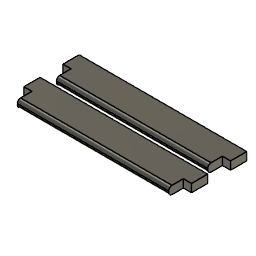
card-shuffler (Autodesk Fusion 360 archive; units mm, degrees)
design "card-shuffler-gates"
part number: 2026-07-29-22-33-21-616
part number: 2026-07-29-22-39-06-031
part number: 2026-07-29-22-39-06-037
Autodesk Fusion 360 part; units mm, degrees
(part 1 of 8)
sketch "Sketch1" plane through (0, 0, 0) normal (0, 0, 1) x (1, 0, 0)
  line L0 (0, 0) -> (93, 0)
  line L1 (93, 0) -> (93, -19)
  line L2 (93, -19) -> (0, -19)
  line L3 (0, -19) -> (0, 0)
  line L4 (0, 0) -> (-5, 0)
  line L5 (-5, 0) -> (-5, -10)
  line L6 (-5, -10) -> (0, -10)
  line L7 (0, -10) -> (0, 0)
  line L8 (93, 0) -> (98, 0)
  line L9 (98, 0) -> (98, -10)
  line L10 (98, -10) -> (93, -10)
  line L11 (93, -10) -> (93, 0)
  dimension "d1" = 93
  dimension "d2" = 19
  constraint horizontal L0
  constraint vertical L1
  constraint horizontal L2
  constraint vertical L3
  constraint coincident L0.start L3.end
  constraint horizontal L4
  constraint vertical L5
  constraint horizontal L6
  constraint vertical L7
  constraint horizontal L8
  constraint vertical L9
  constraint horizontal L10
  constraint vertical L11
  measures "d1" distance of L0.start L0.end
  measures "d2" distance of L0.start L2.end
extrude "Extrude1" add sketch "Sketch1" along normal blind 5 makes body 1
copy_body "CopyPasteBodies1" bodies 1 makes body 2
move_body "Move1" bodies 2 to x (1, 0, 0) y (0, 1, 0) z (0, 0, 1) at (0, 24, 0)
copy_body "Body->Comp1" bodies 1 removing the originals makes body 3 in component "Component"
copy_body "Body->Comp2" bodies 2 removing the originals makes body 4 in component "Component'"
fillet "Fillet1" radius 2 2 edges at (46.5, 5, 0) (46.5, 5, 5) on bodies 4 in component "Component'"
fillet "Fillet1'" radius 2 2 edges at (46.5, -19, 5) (46.5, -19, 0) on bodies 3 in component "Component"
component "Component" placed x (1, 0, 0) y (0, 1, 0) z (0, 0, 1) at (0, 0, 0)
component "Component'" placed x (1, 0, 0) y (0, 1, 0) z (0, 0, 1) at (0, 0, 0)
equation "d2 = 10 mm + 9 mm"

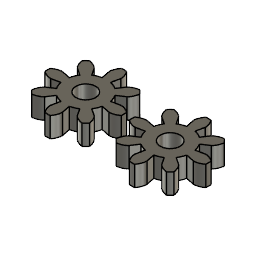
design "card-shuffler-driven-gears"
part number: 2026-07-29-20-17-55-869
part number: 2026-07-29-23-17-52-901
Autodesk Fusion 360 part; units mm, degrees
sketch "Sketch1" plane through (0, 0, 6) normal (0, 0, 1) x (-1, 0, 0)
  arc A0 (-4.7736, 3.1514) -> (-5.6038, 1.147) centre (0, 0) ccw
  line L0 (-5.6038, 1.147) -> (-7.8914, 1.6152)
  line L1 (-7.8914, 1.6152) -> (-7.8925, 1.6154)
  spline S0 degree 5 poles (-7.8925, 1.6154) (-7.8926, 1.6155) (-7.8929, 1.6155) (-7.8933, 1.6156) (-7.8941, 1.6157) (-7.8951, 1.6159) (-7.8964, 1.6161) (-7.8978, 1.6164) (-7.8993, 1.6166) (-7.9011, 1.6169) (-7.9029, 1.6172) (-7.905, 1.6175) (-7.9072, 1.6178) (-7.9095, 1.6181) (-7.912, 1.6184) (-7.9146, 1.6188) (-7.9174, 1.6191) (-7.9204, 1.6195) (-7.9234, 1.6198) (-7.9266, 1.6202) (-7.93, 1.6205) (-7.9334, 1.6209) (-7.9371, 1.6212) (-7.9408, 1.6216) (-7.9447, 1.6219) (-7.9487, 1.6223) (-7.9528, 1.6226) (-7.957, 1.6229) (-7.9614, 1.6232) (-7.9659, 1.6235) (-7.9705, 1.6238) (-7.9752, 1.6241) (-7.9801, 1.6244) (-7.985, 1.6246) (-7.9901, 1.6249) (-7.9953, 1.6251) (-8.0006, 1.6253) (-8.006, 1.6255) (-8.0115, 1.6257) (-8.0171, 1.6258) (-8.0229, 1.6259) (-8.0287, 1.626) (-8.0346, 1.6261) (-8.0407, 1.6262) (-8.0468, 1.6262) (-8.0531, 1.6263) (-8.0594, 1.6263) (-8.0659, 1.6262) (-8.0724, 1.6262) (-8.079, 1.6261) (-8.0858, 1.626) (-8.0926, 1.6258) (-8.0995, 1.6257) (-8.1065, 1.6255) (-8.1136, 1.6253) (-8.1208, 1.625) (-8.1281, 1.6247) (-8.1355, 1.6244) (-8.143, 1.6241) (-8.1505, 1.6237) (-8.1581, 1.6233) (-8.1658, 1.6228) (-8.1737, 1.6223) (-8.1815, 1.6218) (-8.1895, 1.6213) (-8.1976, 1.6207) (-8.2057, 1.6201) (-8.2139, 1.6194) (-8.2222, 1.6187) (-8.2306, 1.618) (-8.239, 1.6172) (-8.2475, 1.6164) (-8.2561, 1.6156) (-8.2648, 1.6147) (-8.2735, 1.6138) (-8.2824, 1.6128) (-8.2913, 1.6118) (-8.3002, 1.6108) (-8.3093, 1.6097) (-8.3184, 1.6086) (-8.3276, 1.6074) (-8.3368, 1.6062) (-8.3461, 1.605) (-8.3555, 1.6037) (-8.365, 1.6024) (-8.3745, 1.601) (-8.3841, 1.5996) (-8.3937, 1.5981) (-8.4035, 1.5966) (-8.4132, 1.5951) (-8.4231, 1.5935) (-8.433, 1.5918) (-8.443, 1.5901) (-8.453, 1.5884) (-8.4631, 1.5866) (-8.4733, 1.5848) (-8.4835, 1.5829) (-8.4938, 1.581) (-8.5041, 1.5791) (-8.5145, 1.577) (-8.525, 1.575) (-8.5355, 1.5729) (-8.546, 1.5707) (-8.5567, 1.5685) (-8.5673, 1.5663) (-8.5781, 1.564) (-8.5889, 1.5616) (-8.5997, 1.5592) (-8.6106, 1.5568) (-8.6215, 1.5543) (-8.6325, 1.5517) (-8.6436, 1.5492) (-8.6547, 1.5465) (-8.6659, 1.5438) (-8.6771, 1.5411) (-8.6883, 1.5383) (-8.6996, 1.5354) (-8.711, 1.5325) (-8.7224, 1.5296) (-8.7338, 1.5266) (-8.7453, 1.5235) (-8.7569, 1.5204) (-8.7684, 1.5173) (-8.7801, 1.514) (-8.7918, 1.5108) (-8.8035, 1.5075) (-8.8153, 1.5041) (-8.8271, 1.5007) (-8.8389, 1.4972) (-8.8508, 1.4937) (-8.8628, 1.4901) (-8.8747, 1.4865) (-8.8868, 1.4828) (-8.8988, 1.479) (-8.9109, 1.4752) (-8.9231, 1.4714) (-8.9353, 1.4675) (-8.9475, 1.4635) (-8.9598, 1.4595) (-8.9721, 1.4554) (-8.9844, 1.4513) (-8.9968, 1.4471) (-9.0092, 1.4429) (-9.0217, 1.4386) (-9.0342, 1.4343) (-9.0467, 1.4299) (-9.0593, 1.4254) (-9.0718, 1.4209) (-9.0845, 1.4163) (-9.0971, 1.4117) (-9.1098, 1.407) (-9.1226, 1.4023) (-9.1353, 1.3975) (-9.1481, 1.3927) (-9.161, 1.3877) (-9.1738, 1.3828) (-9.1867, 1.3778) (-9.1997, 1.3727) (-9.2126, 1.3676) (-9.2256, 1.3624) (-9.2386, 1.3571) (-9.2517, 1.3518) (-9.2647, 1.3465) (-9.2778, 1.3411) (-9.291, 1.3356) (-9.3041, 1.3301) (-9.3173, 1.3245) (-9.3305, 1.3188) (-9.3438, 1.3131) (-9.3571, 1.3074) (-9.3704, 1.3015) (-9.3837, 1.2957) (-9.397, 1.2897) (-9.4104, 1.2837) (-9.4238, 1.2777) (-9.4372, 1.2716) (-9.4507, 1.2654) (-9.4641, 1.2592) (-9.4776, 1.2529) (-9.4911, 1.2465) (-9.5047, 1.2401) (-9.5182, 1.2337) (-9.5318, 1.2272) (-9.5454, 1.2206) (-9.559, 1.214) (-9.5727, 1.2073) (-9.5863, 1.2005) (-9.6, 1.1937) (-9.6137, 1.1868) (-9.6275, 1.1799) (-9.6412, 1.1729) (-9.655, 1.1659) (-9.6687, 1.1588) (-9.6825, 1.1516) (-9.6964, 1.1444) (-9.7102, 1.1371) (-9.7241, 1.1298) (-9.7379, 1.1224) (-9.7518, 1.1149) (-9.7657, 1.1074) (-9.7796, 1.0998) (-9.7936, 1.0922) (-9.8075, 1.0845) (-9.8215, 1.0767) (-9.8355, 1.0689) (-9.8494, 1.061) (-9.8635, 1.0531) (-9.8775, 1.0451) (-9.8915, 1.037) (-9.9056, 1.0289) (-9.9196, 1.0207) (-9.9337, 1.0125) (-9.9478, 1.0042) (-9.9619, 0.9959) (-9.976, 0.9875) (-9.9901, 0.979) (-10.0042, 0.9705) (-10.0184, 0.9619) (-10.0325, 0.9532) (-10.0467, 0.9445) (-10.0608, 0.9357) (-10.075, 0.9269) (-10.0892, 0.918) (-10.1034, 0.9091) (-10.1176, 0.9001) (-10.1318, 0.891) (-10.1461, 0.8819) (-10.1603, 0.8727) (-10.1745, 0.8635) (-10.1888, 0.8542) (-10.203, 0.8448) (-10.2173, 0.8354) (-10.2316, 0.8259) (-10.2458, 0.8163) (-10.2601, 0.8067) (-10.2744, 0.7971) (-10.2887, 0.7874) (-10.303, 0.7776) (-10.3173, 0.7677) (-10.3316, 0.7578) (-10.3459, 0.7479) (-10.3573, 0.7399) (-10.3659, 0.7338) (-10.3716, 0.7298) (-10.3745, 0.7278) knots 0 0 0 0 0 0 0.00416667 0.00833333 0.0125 0.01666667 0.02083333 0.025 0.02916667 0.03333333 0.0375 0.04166667 0.04583333 0.05 0.05416667 0.05833333 0.0625 0.06666667 0.07083333 0.075 0.07916667 0.08333333 0.0875 0.09166667 0.09583333 0.1 0.10416667 0.10833333 0.1125 0.11666667 0.12083333 0.125 0.12916667 0.13333333 0.1375 0.14166667 0.14583333 0.15 0.15416667 0.15833333 0.1625 0.16666667 0.17083333 0.175 0.17916667 0.18333333 0.1875 0.19166667 0.19583333 0.2 0.20416667 0.20833333 0.2125 0.21666667 0.22083333 0.225 0.22916667 0.23333333 0.2375 0.24166667 0.24583333 0.25 0.25416667 0.25833333 0.2625 0.26666667 0.27083333 0.275 0.27916667 0.28333333 0.2875 0.29166667 0.29583333 0.3 0.30416667 0.30833333 0.3125 0.31666667 0.32083333 0.325 0.32916667 0.33333333 0.3375 0.34166667 0.34583333 0.35 0.35416667 0.35833333 0.3625 0.36666667 0.37083333 0.375 0.37916667 0.38333333 0.3875 0.39166667 0.39583333 0.4 0.40416667 0.40833333 0.4125 0.41666667 0.42083333 0.425 0.42916667 0.43333333 0.4375 0.44166667 0.44583333 0.45 0.45416667 0.45833333 0.4625 0.46666667 0.47083333 0.475 0.47916667 0.48333333 0.4875 0.49166667 0.49583333 0.5 0.50416667 0.50833333 0.5125 0.51666667 0.52083333 0.525 0.52916667 0.53333333 0.5375 0.54166667 0.54583333 0.55 0.55416667 0.55833333 0.5625 0.56666667 0.57083333 0.575 0.57916667 0.58333333 0.5875 0.59166667 0.59583333 0.6 0.60416667 0.60833333 0.6125 0.61666667 0.62083333 0.625 0.62916667 0.63333333 0.6375 0.64166667 0.64583333 0.65 0.65416667 0.65833333 0.6625 0.66666667 0.67083333 0.675 0.67916667 0.68333333 0.6875 0.69166667 0.69583333 0.7 0.70416667 0.70833333 0.7125 0.71666667 0.72083333 0.725 0.72916667 0.73333333 0.7375 0.74166667 0.74583333 0.75 0.75416667 0.75833333 0.7625 0.76666667 0.77083333 0.775 0.77916667 0.78333333 0.7875 0.79166667 0.79583333 0.8 0.80416667 0.80833333 0.8125 0.81666667 0.82083333 0.825 0.82916667 0.83333333 0.8375 0.84166667 0.84583333 0.85 0.85416667 0.85833333 0.8625 0.86666667 0.87083333 0.875 0.87916667 0.88333333 0.8875 0.89166667 0.89583333 0.9 0.90416667 0.90833333 0.9125 0.91666667 0.92083333 0.925 0.92916667 0.93333333 0.9375 0.94166667 0.94583333 0.95 0.95416667 0.95833333 0.9625 0.96666667 0.97083333 0.975 0.97916667 0.98333333 0.9875 0.99166667 0.99583333 1 1 1 1 1 1
  arc A1 (-10.3745, 0.7278) -> (-10.3745, -0.7278) centre (0, 0) ccw
  spline S1 degree 5 poles (-10.3745, -0.7278) (-10.3716, -0.7298) (-10.3659, -0.7338) (-10.3573, -0.7399) (-10.3459, -0.7479) (-10.3316, -0.7578) (-10.3173, -0.7677) (-10.303, -0.7776) (-10.2887, -0.7874) (-10.2744, -0.7971) (-10.2601, -0.8067) (-10.2458, -0.8163) (-10.2316, -0.8259) (-10.2173, -0.8354) (-10.203, -0.8448) (-10.1888, -0.8542) (-10.1745, -0.8635) (-10.1603, -0.8727) (-10.1461, -0.8819) (-10.1318, -0.891) (-10.1176, -0.9001) (-10.1034, -0.9091) (-10.0892, -0.918) (-10.075, -0.9269) (-10.0608, -0.9357) (-10.0467, -0.9445) (-10.0325, -0.9532) (-10.0184, -0.9619) (-10.0042, -0.9705) (-9.9901, -0.979) (-9.976, -0.9875) (-9.9619, -0.9959) (-9.9478, -1.0042) (-9.9337, -1.0125) (-9.9196, -1.0207) (-9.9056, -1.0289) (-9.8915, -1.037) (-9.8775, -1.0451) (-9.8635, -1.0531) (-9.8494, -1.061) (-9.8355, -1.0689) (-9.8215, -1.0767) (-9.8075, -1.0845) (-9.7936, -1.0922) (-9.7796, -1.0998) (-9.7657, -1.1074) (-9.7518, -1.1149) (-9.7379, -1.1224) (-9.7241, -1.1298) (-9.7102, -1.1371) (-9.6964, -1.1444) (-9.6825, -1.1516) (-9.6687, -1.1588) (-9.655, -1.1659) (-9.6412, -1.1729) (-9.6275, -1.1799) (-9.6137, -1.1868) (-9.6, -1.1937) (-9.5863, -1.2005) (-9.5727, -1.2073) (-9.559, -1.214) (-9.5454, -1.2206) (-9.5318, -1.2272) (-9.5182, -1.2337) (-9.5047, -1.2401) (-9.4911, -1.2465) (-9.4776, -1.2529) (-9.4641, -1.2592) (-9.4507, -1.2654) (-9.4372, -1.2716) (-9.4238, -1.2777) (-9.4104, -1.2837) (-9.397, -1.2897) (-9.3837, -1.2957) (-9.3704, -1.3015) (-9.3571, -1.3074) (-9.3438, -1.3131) (-9.3305, -1.3188) (-9.3173, -1.3245) (-9.3041, -1.3301) (-9.291, -1.3356) (-9.2778, -1.3411) (-9.2647, -1.3465) (-9.2517, -1.3518) (-9.2386, -1.3571) (-9.2256, -1.3624) (-9.2126, -1.3676) (-9.1997, -1.3727) (-9.1867, -1.3778) (-9.1738, -1.3828) (-9.161, -1.3877) (-9.1481, -1.3927) (-9.1353, -1.3975) (-9.1226, -1.4023) (-9.1098, -1.407) (-9.0971, -1.4117) (-9.0845, -1.4163) (-9.0718, -1.4209) (-9.0593, -1.4254) (-9.0467, -1.4299) (-9.0342, -1.4343) (-9.0217, -1.4386) (-9.0092, -1.4429) (-8.9968, -1.4471) (-8.9844, -1.4513) (-8.9721, -1.4554) (-8.9598, -1.4595) (-8.9475, -1.4635) (-8.9353, -1.4675) (-8.9231, -1.4714) (-8.9109, -1.4752) (-8.8988, -1.479) (-8.8868, -1.4828) (-8.8747, -1.4865) (-8.8628, -1.4901) (-8.8508, -1.4937) (-8.8389, -1.4972) (-8.8271, -1.5007) (-8.8153, -1.5041) (-8.8035, -1.5075) (-8.7918, -1.5108) (-8.7801, -1.514) (-8.7684, -1.5173) (-8.7569, -1.5204) (-8.7453, -1.5235) (-8.7338, -1.5266) (-8.7224, -1.5296) (-8.711, -1.5325) (-8.6996, -1.5354) (-8.6883, -1.5383) (-8.6771, -1.5411) (-8.6659, -1.5438) (-8.6547, -1.5465) (-8.6436, -1.5492) (-8.6325, -1.5517) (-8.6215, -1.5543) (-8.6106, -1.5568) (-8.5997, -1.5592) (-8.5889, -1.5616) (-8.5781, -1.564) (-8.5673, -1.5663) (-8.5567, -1.5685) (-8.546, -1.5707) (-8.5355, -1.5729) (-8.525, -1.575) (-8.5145, -1.577) (-8.5041, -1.5791) (-8.4938, -1.581) (-8.4835, -1.5829) (-8.4733, -1.5848) (-8.4631, -1.5866) (-8.453, -1.5884) (-8.443, -1.5901) (-8.433, -1.5918) (-8.4231, -1.5935) (-8.4132, -1.5951) (-8.4035, -1.5966) (-8.3937, -1.5981) (-8.3841, -1.5996) (-8.3745, -1.601) (-8.365, -1.6024) (-8.3555, -1.6037) (-8.3461, -1.605) (-8.3368, -1.6062) (-8.3276, -1.6074) (-8.3184, -1.6086) (-8.3093, -1.6097) (-8.3002, -1.6108) (-8.2913, -1.6118) (-8.2824, -1.6128) (-8.2735, -1.6138) (-8.2648, -1.6147) (-8.2561, -1.6156) (-8.2475, -1.6164) (-8.239, -1.6172) (-8.2306, -1.618) (-8.2222, -1.6187) (-8.2139, -1.6194) (-8.2057, -1.6201) (-8.1976, -1.6207) (-8.1895, -1.6213) (-8.1815, -1.6218) (-8.1737, -1.6223) (-8.1658, -1.6228) (-8.1581, -1.6233) (-8.1505, -1.6237) (-8.143, -1.6241) (-8.1355, -1.6244) (-8.1281, -1.6247) (-8.1208, -1.625) (-8.1136, -1.6253) (-8.1065, -1.6255) (-8.0995, -1.6257) (-8.0926, -1.6258) (-8.0858, -1.626) (-8.079, -1.6261) (-8.0724, -1.6262) (-8.0659, -1.6262) (-8.0594, -1.6263) (-8.0531, -1.6263) (-8.0468, -1.6262) (-8.0407, -1.6262) (-8.0346, -1.6261) (-8.0287, -1.626) (-8.0229, -1.6259) (-8.0171, -1.6258) (-8.0115, -1.6257) (-8.006, -1.6255) (-8.0006, -1.6253) (-7.9953, -1.6251) (-7.9901, -1.6249) (-7.985, -1.6246) (-7.9801, -1.6244) (-7.9752, -1.6241) (-7.9705, -1.6238) (-7.9659, -1.6235) (-7.9614, -1.6232) (-7.957, -1.6229) (-7.9528, -1.6226) (-7.9487, -1.6223) (-7.9447, -1.6219) (-7.9408, -1.6216) (-7.9371, -1.6212) (-7.9334, -1.6209) (-7.93, -1.6205) (-7.9266, -1.6202) (-7.9234, -1.6198) (-7.9204, -1.6195) (-7.9174, -1.6191) (-7.9146, -1.6188) (-7.912, -1.6184) (-7.9095, -1.6181) (-7.9072, -1.6178) (-7.905, -1.6175) (-7.9029, -1.6172) (-7.9011, -1.6169) (-7.8993, -1.6166) (-7.8978, -1.6164) (-7.8964, -1.6161) (-7.8951, -1.6159) (-7.8941, -1.6157) (-7.8933, -1.6156) (-7.8929, -1.6155) (-7.8926, -1.6155) (-7.8925, -1.6154) knots -1 -1 -1 -1 -1 -1 -0.99583333 -0.99166667 -0.9875 -0.98333333 -0.97916667 -0.975 -0.97083333 -0.96666667 -0.9625 -0.95833333 -0.95416667 -0.95 -0.94583333 -0.94166667 -0.9375 -0.93333333 -0.92916667 -0.925 -0.92083333 -0.91666667 -0.9125 -0.90833333 -0.90416667 -0.9 -0.89583333 -0.89166667 -0.8875 -0.88333333 -0.87916667 -0.875 -0.87083333 -0.86666667 -0.8625 -0.85833333 -0.85416667 -0.85 -0.84583333 -0.84166667 -0.8375 -0.83333333 -0.82916667 -0.825 -0.82083333 -0.81666667 -0.8125 -0.80833333 -0.80416667 -0.8 -0.79583333 -0.79166667 -0.7875 -0.78333333 -0.77916667 -0.775 -0.77083333 -0.76666667 -0.7625 -0.75833333 -0.75416667 -0.75 -0.74583333 -0.74166667 -0.7375 -0.73333333 -0.72916667 -0.725 -0.72083333 -0.71666667 -0.7125 -0.70833333 -0.70416667 -0.7 -0.69583333 -0.69166667 -0.6875 -0.68333333 -0.67916667 -0.675 -0.67083333 -0.66666667 -0.6625 -0.65833333 -0.65416667 -0.65 -0.64583333 -0.64166667 -0.6375 -0.63333333 -0.62916667 -0.625 -0.62083333 -0.61666667 -0.6125 -0.60833333 -0.60416667 -0.6 -0.59583333 -0.59166667 -0.5875 -0.58333333 -0.57916667 -0.575 -0.57083333 -0.56666667 -0.5625 -0.55833333 -0.55416667 -0.55 -0.54583333 -0.54166667 -0.5375 -0.53333333 -0.52916667 -0.525 -0.52083333 -0.51666667 -0.5125 -0.50833333 -0.50416667 -0.5 -0.49583333 -0.49166667 -0.4875 -0.48333333 -0.47916667 -0.475 -0.47083333 -0.46666667 -0.4625 -0.45833333 -0.45416667 -0.45 -0.44583333 -0.44166667 -0.4375 -0.43333333 -0.42916667 -0.425 -0.42083333 -0.41666667 -0.4125 -0.40833333 -0.40416667 -0.4 -0.39583333 -0.39166667 -0.3875 -0.38333333 -0.37916667 -0.375 -0.37083333 -0.36666667 -0.3625 -0.35833333 -0.35416667 -0.35 -0.34583333 -0.34166667 -0.3375 -0.33333333 -0.32916667 -0.325 -0.32083333 -0.31666667 -0.3125 -0.30833333 -0.30416667 -0.3 -0.29583333 -0.29166667 -0.2875 -0.28333333 -0.27916667 -0.275 -0.27083333 -0.26666667 -0.2625 -0.25833333 -0.25416667 -0.25 -0.24583333 -0.24166667 -0.2375 -0.23333333 -0.22916667 -0.225 -0.22083333 -0.21666667 -0.2125 -0.20833333 -0.20416667 -0.2 -0.19583333 -0.19166667 -0.1875 -0.18333333 -0.17916667 -0.175 -0.17083333 -0.16666667 -0.1625 -0.15833333 -0.15416667 -0.15 -0.14583333 -0.14166667 -0.1375 -0.13333333 -0.12916667 -0.125 -0.12083333 -0.11666667 -0.1125 -0.10833333 -0.10416667 -0.1 -0.09583333 -0.09166667 -0.0875 -0.08333333 -0.07916667 -0.075 -0.07083333 -0.06666667 -0.0625 -0.05833333 -0.05416667 -0.05 -0.04583333 -0.04166667 -0.0375 -0.03333333 -0.02916667 -0.025 -0.02083333 -0.01666667 -0.0125 -0.00833333 -0.00416667 0 0 0 0 0 0
  line L2 (-7.8925, -1.6154) -> (-7.8914, -1.6152)
  line L3 (-7.8914, -1.6152) -> (-5.6038, -1.147)
  arc A2 (-5.6038, -1.147) -> (-4.7736, -3.1514) centre (0, 0) ccw
  line L4 (-4.7736, -3.1514) -> (-6.7222, -4.4379)
  line L5 (-6.7222, -4.4379) -> (-6.7231, -4.4385)
  spline S2 degree 5 poles (-6.7231, -4.4385) (-6.7232, -4.4386) (-6.7235, -4.4388) (-6.7238, -4.439) (-6.7244, -4.4394) (-6.7253, -4.4401) (-6.7263, -4.4408) (-6.7275, -4.4416) (-6.7288, -4.4425) (-6.7302, -4.4436) (-6.7317, -4.4447) (-6.7334, -4.4459) (-6.7352, -4.4473) (-6.737, -4.4487) (-6.739, -4.4502) (-6.7411, -4.4519) (-6.7434, -4.4536) (-6.7457, -4.4554) (-6.7481, -4.4573) (-6.7506, -4.4593) (-6.7532, -4.4614) (-6.7559, -4.4637) (-6.7587, -4.466) (-6.7616, -4.4684) (-6.7646, -4.4708) (-6.7677, -4.4734) (-6.7708, -4.4761) (-6.774, -4.4789) (-6.7774, -4.4818) (-6.7807, -4.4847) (-6.7842, -4.4878) (-6.7877, -4.4909) (-6.7914, -4.4942) (-6.7951, -4.4975) (-6.7988, -4.5009) (-6.8026, -4.5044) (-6.8065, -4.508) (-6.8105, -4.5117) (-6.8145, -4.5155) (-6.8186, -4.5194) (-6.8227, -4.5233) (-6.8269, -4.5274) (-6.8312, -4.5315) (-6.8355, -4.5357) (-6.8399, -4.54) (-6.8443, -4.5444) (-6.8488, -4.5489) (-6.8533, -4.5535) (-6.8579, -4.5582) (-6.8626, -4.5629) (-6.8672, -4.5678) (-6.872, -4.5727) (-6.8768, -4.5777) (-6.8816, -4.5828) (-6.8864, -4.588) (-6.8914, -4.5932) (-6.8963, -4.5986) (-6.9013, -4.604) (-6.9063, -4.6096) (-6.9114, -4.6152) (-6.9165, -4.6208) (-6.9216, -4.6266) (-6.9268, -4.6325) (-6.932, -4.6384) (-6.9373, -4.6444) (-6.9426, -4.6505) (-6.9479, -4.6567) (-6.9532, -4.663) (-6.9586, -4.6693) (-6.964, -4.6758) (-6.9694, -4.6823) (-6.9749, -4.6889) (-6.9804, -4.6956) (-6.9859, -4.7023) (-6.9914, -4.7092) (-6.997, -4.7161) (-7.0025, -4.7231) (-7.0082, -4.7301) (-7.0138, -4.7373) (-7.0194, -4.7445) (-7.0251, -4.7518) (-7.0308, -4.7592) (-7.0365, -4.7667) (-7.0422, -4.7743) (-7.048, -4.7819) (-7.0537, -4.7896) (-7.0595, -4.7974) (-7.0653, -4.8052) (-7.0711, -4.8132) (-7.0769, -4.8212) (-7.0828, -4.8293) (-7.0886, -4.8375) (-7.0945, -4.8457) (-7.1004, -4.854) (-7.1062, -4.8624) (-7.1121, -4.8709) (-7.118, -4.8794) (-7.1239, -4.8881) (-7.1299, -4.8968) (-7.1358, -4.9055) (-7.1417, -4.9144) (-7.1477, -4.9233) (-7.1536, -4.9323) (-7.1596, -4.9414) (-7.1655, -4.9505) (-7.1715, -4.9597) (-7.1775, -4.969) (-7.1834, -4.9784) (-7.1894, -4.9878) (-7.1954, -4.9973) (-7.2014, -5.0069) (-7.2074, -5.0165) (-7.2133, -5.0262) (-7.2193, -5.036) (-7.2253, -5.0459) (-7.2313, -5.0558) (-7.2373, -5.0658) (-7.2432, -5.0759) (-7.2492, -5.0861) (-7.2552, -5.0963) (-7.2612, -5.1066) (-7.2671, -5.1169) (-7.2731, -5.1274) (-7.279, -5.1379) (-7.285, -5.1484) (-7.2909, -5.1591) (-7.2969, -5.1698) (-7.3028, -5.1805) (-7.3087, -5.1914) (-7.3147, -5.2023) (-7.3206, -5.2133) (-7.3265, -5.2243) (-7.3324, -5.2354) (-7.3383, -5.2466) (-7.3441, -5.2578) (-7.35, -5.2692) (-7.3559, -5.2805) (-7.3617, -5.292) (-7.3675, -5.3035) (-7.3734, -5.3151) (-7.3792, -5.3267) (-7.385, -5.3384) (-7.3908, -5.3502) (-7.3965, -5.362) (-7.4023, -5.3739) (-7.408, -5.3859) (-7.4138, -5.3979) (-7.4195, -5.41) (-7.4252, -5.4222) (-7.4309, -5.4344) (-7.4366, -5.4467) (-7.4422, -5.4591) (-7.4478, -5.4715) (-7.4535, -5.484) (-7.4591, -5.4965) (-7.4647, -5.5091) (-7.4702, -5.5218) (-7.4758, -5.5345) (-7.4813, -5.5473) (-7.4868, -5.5601) (-7.4923, -5.5731) (-7.4978, -5.586) (-7.5033, -5.5991) (-7.5087, -5.6122) (-7.5141, -5.6253) (-7.5195, -5.6385) (-7.5249, -5.6518) (-7.5302, -5.6651) (-7.5356, -5.6785) (-7.5409, -5.692) (-7.5462, -5.7055) (-7.5514, -5.7191) (-7.5567, -5.7327) (-7.5619, -5.7464) (-7.5671, -5.7602) (-7.5722, -5.774) (-7.5774, -5.7878) (-7.5825, -5.8018) (-7.5876, -5.8158) (-7.5927, -5.8298) (-7.5977, -5.8439) (-7.6028, -5.8581) (-7.6077, -5.8723) (-7.6127, -5.8865) (-7.6177, -5.9009) (-7.6226, -5.9152) (-7.6275, -5.9297) (-7.6323, -5.9442) (-7.6372, -5.9587) (-7.642, -5.9733) (-7.6467, -5.988) (-7.6515, -6.0027) (-7.6562, -6.0175) (-7.6609, -6.0323) (-7.6656, -6.0472) (-7.6702, -6.0621) (-7.6748, -6.0771) (-7.6794, -6.0921) (-7.6839, -6.1072) (-7.6884, -6.1224) (-7.6929, -6.1376) (-7.6974, -6.1528) (-7.7018, -6.1681) (-7.7062, -6.1835) (-7.7105, -6.1989) (-7.7149, -6.2144) (-7.7192, -6.2299) (-7.7234, -6.2454) (-7.7276, -6.2611) (-7.7318, -6.2767) (-7.736, -6.2925) (-7.7401, -6.3082) (-7.7442, -6.324) (-7.7483, -6.3399) (-7.7523, -6.3558) (-7.7563, -6.3718) (-7.7603, -6.3878) (-7.7642, -6.4039) (-7.7681, -6.42) (-7.7719, -6.4362) (-7.7758, -6.4524) (-7.7796, -6.4687) (-7.7833, -6.485) (-7.787, -6.5014) (-7.7907, -6.5178) (-7.7943, -6.5343) (-7.7979, -6.5508) (-7.8015, -6.5673) (-7.805, -6.5839) (-7.8085, -6.6006) (-7.812, -6.6173) (-7.8154, -6.634) (-7.8188, -6.6508) (-7.8221, -6.6677) (-7.8254, -6.6845) (-7.8287, -6.7015) (-7.8319, -6.7185) (-7.8351, -6.7355) (-7.8383, -6.7525) (-7.8414, -6.7697) (-7.8445, -6.7868) (-7.8469, -6.8006) (-7.8487, -6.8109) (-7.8499, -6.8178) (-7.8505, -6.8213) knots 0 0 0 0 0 0 0.00416667 0.00833333 0.0125 0.01666667 0.02083333 0.025 0.02916667 0.03333333 0.0375 0.04166667 0.04583333 0.05 0.05416667 0.05833333 0.0625 0.06666667 0.07083333 0.075 0.07916667 0.08333333 0.0875 0.09166667 0.09583333 0.1 0.10416667 0.10833333 0.1125 0.11666667 0.12083333 0.125 0.12916667 0.13333333 0.1375 0.14166667 0.14583333 0.15 0.15416667 0.15833333 0.1625 0.16666667 0.17083333 0.175 0.17916667 0.18333333 0.1875 0.19166667 0.19583333 0.2 0.20416667 0.20833333 0.2125 0.21666667 0.22083333 0.225 0.22916667 0.23333333 0.2375 0.24166667 0.24583333 0.25 0.25416667 0.25833333 0.2625 0.26666667 0.27083333 0.275 0.27916667 0.28333333 0.2875 0.29166667 0.29583333 0.3 0.30416667 0.30833333 0.3125 0.31666667 0.32083333 0.325 0.32916667 0.33333333 0.3375 0.34166667 0.34583333 0.35 0.35416667 0.35833333 0.3625 0.36666667 0.37083333 0.375 0.37916667 0.38333333 0.3875 0.39166667 0.39583333 0.4 0.40416667 0.40833333 0.4125 0.41666667 0.42083333 0.425 0.42916667 0.43333333 0.4375 0.44166667 0.44583333 0.45 0.45416667 0.45833333 0.4625 0.46666667 0.47083333 0.475 0.47916667 0.48333333 0.4875 0.49166667 0.49583333 0.5 0.50416667 0.50833333 0.5125 0.51666667 0.52083333 0.525 0.52916667 0.53333333 0.5375 0.54166667 0.54583333 0.55 0.55416667 0.55833333 0.5625 0.56666667 0.57083333 0.575 0.57916667 0.58333333 0.5875 0.59166667 0.59583333 0.6 0.60416667 0.60833333 0.6125 0.61666667 0.62083333 0.625 0.62916667 0.63333333 0.6375 0.64166667 0.64583333 0.65 0.65416667 0.65833333 0.6625 0.66666667 0.67083333 0.675 0.67916667 0.68333333 0.6875 0.69166667 0.69583333 0.7 0.70416667 0.70833333 0.7125 0.71666667 0.72083333 0.725 0.72916667 0.73333333 0.7375 0.74166667 0.74583333 0.75 0.75416667 0.75833333 0.7625 0.76666667 0.77083333 0.775 0.77916667 0.78333333 0.7875 0.79166667 0.79583333 0.8 0.80416667 0.80833333 0.8125 0.81666667 0.82083333 0.825 0.82916667 0.83333333 0.8375 0.84166667 0.84583333 0.85 0.85416667 0.85833333 0.8625 0.86666667 0.87083333 0.875 0.87916667 0.88333333 0.8875 0.89166667 0.89583333 0.9 0.90416667 0.90833333 0.9125 0.91666667 0.92083333 0.925 0.92916667 0.93333333 0.9375 0.94166667 0.94583333 0.95 0.95416667 0.95833333 0.9625 0.96666667 0.97083333 0.975 0.97916667 0.98333333 0.9875 0.99166667 0.99583333 1 1 1 1 1 1
  arc A3 (-7.8505, -6.8213) -> (-6.8213, -7.8505) centre (0, 0) ccw
  spline S3 degree 5 poles (-6.8213, -7.8505) (-6.8178, -7.8499) (-6.8109, -7.8487) (-6.8006, -7.8469) (-6.7868, -7.8445) (-6.7697, -7.8414) (-6.7525, -7.8383) (-6.7355, -7.8351) (-6.7185, -7.8319) (-6.7015, -7.8287) (-6.6845, -7.8254) (-6.6677, -7.8221) (-6.6508, -7.8188) (-6.634, -7.8154) (-6.6173, -7.812) (-6.6006, -7.8085) (-6.5839, -7.805) (-6.5673, -7.8015) (-6.5508, -7.7979) (-6.5343, -7.7943) (-6.5178, -7.7907) (-6.5014, -7.787) (-6.485, -7.7833) (-6.4687, -7.7796) (-6.4524, -7.7758) (-6.4362, -7.7719) (-6.42, -7.7681) (-6.4039, -7.7642) (-6.3878, -7.7603) (-6.3718, -7.7563) (-6.3558, -7.7523) (-6.3399, -7.7483) (-6.324, -7.7442) (-6.3082, -7.7401) (-6.2925, -7.736) (-6.2767, -7.7318) (-6.2611, -7.7276) (-6.2454, -7.7234) (-6.2299, -7.7192) (-6.2144, -7.7149) (-6.1989, -7.7105) (-6.1835, -7.7062) (-6.1681, -7.7018) (-6.1528, -7.6974) (-6.1376, -7.6929) (-6.1224, -7.6884) (-6.1072, -7.6839) (-6.0921, -7.6794) (-6.0771, -7.6748) (-6.0621, -7.6702) (-6.0472, -7.6656) (-6.0323, -7.6609) (-6.0175, -7.6562) (-6.0027, -7.6515) (-5.988, -7.6467) (-5.9733, -7.642) (-5.9587, -7.6372) (-5.9442, -7.6323) (-5.9297, -7.6275) (-5.9152, -7.6226) (-5.9009, -7.6177) (-5.8865, -7.6127) (-5.8723, -7.6077) (-5.8581, -7.6028) (-5.8439, -7.5977) (-5.8298, -7.5927) (-5.8158, -7.5876) (-5.8018, -7.5825) (-5.7878, -7.5774) (-5.774, -7.5722) (-5.7602, -7.5671) (-5.7464, -7.5619) (-5.7327, -7.5567) (-5.7191, -7.5514) (-5.7055, -7.5462) (-5.692, -7.5409) (-5.6785, -7.5356) (-5.6651, -7.5302) (-5.6518, -7.5249) (-5.6385, -7.5195) (-5.6253, -7.5141) (-5.6122, -7.5087) (-5.5991, -7.5033) (-5.586, -7.4978) (-5.5731, -7.4923) (-5.5601, -7.4868) (-5.5473, -7.4813) (-5.5345, -7.4758) (-5.5218, -7.4702) (-5.5091, -7.4647) (-5.4965, -7.4591) (-5.484, -7.4535) (-5.4715, -7.4478) (-5.4591, -7.4422) (-5.4467, -7.4366) (-5.4344, -7.4309) (-5.4222, -7.4252) (-5.41, -7.4195) (-5.3979, -7.4138) (-5.3859, -7.408) (-5.3739, -7.4023) (-5.362, -7.3965) (-5.3502, -7.3908) (-5.3384, -7.385) (-5.3267, -7.3792) (-5.3151, -7.3734) (-5.3035, -7.3675) (-5.292, -7.3617) (-5.2805, -7.3559) (-5.2692, -7.35) (-5.2578, -7.3441) (-5.2466, -7.3383) (-5.2354, -7.3324) (-5.2243, -7.3265) (-5.2133, -7.3206) (-5.2023, -7.3147) (-5.1914, -7.3087) (-5.1805, -7.3028) (-5.1698, -7.2969) (-5.1591, -7.2909) (-5.1484, -7.285) (-5.1379, -7.279) (-5.1274, -7.2731) (-5.1169, -7.2671) (-5.1066, -7.2612) (-5.0963, -7.2552) (-5.0861, -7.2492) (-5.0759, -7.2432) (-5.0658, -7.2373) (-5.0558, -7.2313) (-5.0459, -7.2253) (-5.036, -7.2193) (-5.0262, -7.2133) (-5.0165, -7.2074) (-5.0069, -7.2014) (-4.9973, -7.1954) (-4.9878, -7.1894) (-4.9784, -7.1834) (-4.969, -7.1775) (-4.9597, -7.1715) (-4.9505, -7.1655) (-4.9414, -7.1596) (-4.9323, -7.1536) (-4.9233, -7.1477) (-4.9144, -7.1417) (-4.9055, -7.1358) (-4.8968, -7.1299) (-4.8881, -7.1239) (-4.8794, -7.118) (-4.8709, -7.1121) (-4.8624, -7.1062) (-4.854, -7.1004) (-4.8457, -7.0945) (-4.8375, -7.0886) (-4.8293, -7.0828) (-4.8212, -7.0769) (-4.8132, -7.0711) (-4.8052, -7.0653) (-4.7974, -7.0595) (-4.7896, -7.0537) (-4.7819, -7.048) (-4.7743, -7.0422) (-4.7667, -7.0365) (-4.7592, -7.0308) (-4.7518, -7.0251) (-4.7445, -7.0194) (-4.7373, -7.0138) (-4.7301, -7.0082) (-4.7231, -7.0025) (-4.7161, -6.997) (-4.7092, -6.9914) (-4.7023, -6.9859) (-4.6956, -6.9804) (-4.6889, -6.9749) (-4.6823, -6.9694) (-4.6758, -6.964) (-4.6693, -6.9586) (-4.663, -6.9532) (-4.6567, -6.9479) (-4.6505, -6.9426) (-4.6444, -6.9373) (-4.6384, -6.932) (-4.6325, -6.9268) (-4.6266, -6.9216) (-4.6208, -6.9165) (-4.6152, -6.9114) (-4.6096, -6.9063) (-4.604, -6.9013) (-4.5986, -6.8963) (-4.5932, -6.8914) (-4.588, -6.8864) (-4.5828, -6.8816) (-4.5777, -6.8768) (-4.5727, -6.872) (-4.5678, -6.8672) (-4.5629, -6.8626) (-4.5582, -6.8579) (-4.5535, -6.8533) (-4.5489, -6.8488) (-4.5444, -6.8443) (-4.54, -6.8399) (-4.5357, -6.8355) (-4.5315, -6.8312) (-4.5274, -6.8269) (-4.5233, -6.8227) (-4.5194, -6.8186) (-4.5155, -6.8145) (-4.5117, -6.8105) (-4.508, -6.8065) (-4.5044, -6.8026) (-4.5009, -6.7988) (-4.4975, -6.7951) (-4.4942, -6.7914) (-4.4909, -6.7877) (-4.4878, -6.7842) (-4.4847, -6.7807) (-4.4818, -6.7774) (-4.4789, -6.774) (-4.4761, -6.7708) (-4.4734, -6.7677) (-4.4708, -6.7646) (-4.4684, -6.7616) (-4.466, -6.7587) (-4.4637, -6.7559) (-4.4614, -6.7532) (-4.4593, -6.7506) (-4.4573, -6.7481) (-4.4554, -6.7457) (-4.4536, -6.7434) (-4.4519, -6.7411) (-4.4502, -6.739) (-4.4487, -6.737) (-4.4473, -6.7352) (-4.4459, -6.7334) (-4.4447, -6.7317) (-4.4436, -6.7302) (-4.4425, -6.7288) (-4.4416, -6.7275) (-4.4408, -6.7263) (-4.4401, -6.7253) (-4.4394, -6.7244) (-4.439, -6.7238) (-4.4388, -6.7235) (-4.4386, -6.7232) (-4.4385, -6.7231) knots -1 -1 -1 -1 -1 -1 -0.99583333 -0.99166667 -0.9875 -0.98333333 -0.97916667 -0.975 -0.97083333 -0.96666667 -0.9625 -0.95833333 -0.95416667 -0.95 -0.94583333 -0.94166667 -0.9375 -0.93333333 -0.92916667 -0.925 -0.92083333 -0.91666667 -0.9125 -0.90833333 -0.90416667 -0.9 -0.89583333 -0.89166667 -0.8875 -0.88333333 -0.87916667 -0.875 -0.87083333 -0.86666667 -0.8625 -0.85833333 -0.85416667 -0.85 -0.84583333 -0.84166667 -0.8375 -0.83333333 -0.82916667 -0.825 -0.82083333 -0.81666667 -0.8125 -0.80833333 -0.80416667 -0.8 -0.79583333 -0.79166667 -0.7875 -0.78333333 -0.77916667 -0.775 -0.77083333 -0.76666667 -0.7625 -0.75833333 -0.75416667 -0.75 -0.74583333 -0.74166667 -0.7375 -0.73333333 -0.72916667 -0.725 -0.72083333 -0.71666667 -0.7125 -0.70833333 -0.70416667 -0.7 -0.69583333 -0.69166667 -0.6875 -0.68333333 -0.67916667 -0.675 -0.67083333 -0.66666667 -0.6625 -0.65833333 -0.65416667 -0.65 -0.64583333 -0.64166667 -0.6375 -0.63333333 -0.62916667 -0.625 -0.62083333 -0.61666667 -0.6125 -0.60833333 -0.60416667 -0.6 -0.59583333 -0.59166667 -0.5875 -0.58333333 -0.57916667 -0.575 -0.57083333 -0.56666667 -0.5625 -0.55833333 -0.55416667 -0.55 -0.54583333 -0.54166667 -0.5375 -0.53333333 -0.52916667 -0.525 -0.52083333 -0.51666667 -0.5125 -0.50833333 -0.50416667 -0.5 -0.49583333 -0.49166667 -0.4875 -0.48333333 -0.47916667 -0.475 -0.47083333 -0.46666667 -0.4625 -0.45833333 -0.45416667 -0.45 -0.44583333 -0.44166667 -0.4375 -0.43333333 -0.42916667 -0.425 -0.42083333 -0.41666667 -0.4125 -0.40833333 -0.40416667 -0.4 -0.39583333 -0.39166667 -0.3875 -0.38333333 -0.37916667 -0.375 -0.37083333 -0.36666667 -0.3625 -0.35833333 -0.35416667 -0.35 -0.34583333 -0.34166667 -0.3375 -0.33333333 -0.32916667 -0.325 -0.32083333 -0.31666667 -0.3125 -0.30833333 -0.30416667 -0.3 -0.29583333 -0.29166667 -0.2875 -0.28333333 -0.27916667 -0.275 -0.27083333 -0.26666667 -0.2625 -0.25833333 -0.25416667 -0.25 -0.24583333 -0.24166667 -0.2375 -0.23333333 -0.22916667 -0.225 -0.22083333 -0.21666667 -0.2125 -0.20833333 -0.20416667 -0.2 -0.19583333 -0.19166667 -0.1875 -0.18333333 -0.17916667 -0.175 -0.17083333 -0.16666667 -0.1625 -0.15833333 -0.15416667 -0.15 -0.14583333 -0.14166667 -0.1375 -0.13333333 -0.12916667 -0.125 -0.12083333 -0.11666667 -0.1125 -0.10833333 -0.10416667 -0.1 -0.09583333 -0.09166667 -0.0875 -0.08333333 -0.07916667 -0.075 -0.07083333 -0.06666667 -0.0625 -0.05833333 -0.05416667 -0.05 -0.04583333 -0.04166667 -0.0375 -0.03333333 -0.02916667 -0.025 -0.02083333 -0.01666667 -0.0125 -0.00833333 -0.00416667 0 0 0 0 0 0
  line L6 (-4.4385, -6.7231) -> (-4.4379, -6.7222)
  line L7 (-4.4379, -6.7222) -> (-3.1514, -4.7736)
  arc A4 (-3.1514, -4.7736) -> (-1.147, -5.6038) centre (0, 0) ccw
  line L8 (-1.147, -5.6038) -> (-1.6152, -7.8914)
  line L9 (-1.6152, -7.8914) -> (-1.6154, -7.8925)
  spline S4 degree 5 poles (-1.6154, -7.8925) (-1.6155, -7.8926) (-1.6155, -7.8929) (-1.6156, -7.8933) (-1.6157, -7.8941) (-1.6159, -7.8951) (-1.6161, -7.8964) (-1.6164, -7.8978) (-1.6166, -7.8993) (-1.6169, -7.9011) (-1.6172, -7.9029) (-1.6175, -7.905) (-1.6178, -7.9072) (-1.6181, -7.9095) (-1.6184, -7.912) (-1.6188, -7.9146) (-1.6191, -7.9174) (-1.6195, -7.9204) (-1.6198, -7.9234) (-1.6202, -7.9266) (-1.6205, -7.93) (-1.6209, -7.9334) (-1.6212, -7.9371) (-1.6216, -7.9408) (-1.6219, -7.9447) (-1.6223, -7.9487) (-1.6226, -7.9528) (-1.6229, -7.957) (-1.6232, -7.9614) (-1.6235, -7.9659) (-1.6238, -7.9705) (-1.6241, -7.9752) (-1.6244, -7.9801) (-1.6246, -7.985) (-1.6249, -7.9901) (-1.6251, -7.9953) (-1.6253, -8.0006) (-1.6255, -8.006) (-1.6257, -8.0115) (-1.6258, -8.0171) (-1.6259, -8.0229) (-1.626, -8.0287) (-1.6261, -8.0346) (-1.6262, -8.0407) (-1.6262, -8.0468) (-1.6263, -8.0531) (-1.6263, -8.0594) (-1.6262, -8.0659) (-1.6262, -8.0724) (-1.6261, -8.079) (-1.626, -8.0858) (-1.6258, -8.0926) (-1.6257, -8.0995) (-1.6255, -8.1065) (-1.6253, -8.1136) (-1.625, -8.1208) (-1.6247, -8.1281) (-1.6244, -8.1355) (-1.6241, -8.143) (-1.6237, -8.1505) (-1.6233, -8.1581) (-1.6228, -8.1658) (-1.6223, -8.1737) (-1.6218, -8.1815) (-1.6213, -8.1895) (-1.6207, -8.1976) (-1.6201, -8.2057) (-1.6194, -8.2139) (-1.6187, -8.2222) (-1.618, -8.2306) (-1.6172, -8.239) (-1.6164, -8.2475) (-1.6156, -8.2561) (-1.6147, -8.2648) (-1.6138, -8.2735) (-1.6128, -8.2824) (-1.6118, -8.2913) (-1.6108, -8.3002) (-1.6097, -8.3093) (-1.6086, -8.3184) (-1.6074, -8.3276) (-1.6062, -8.3368) (-1.605, -8.3461) (-1.6037, -8.3555) (-1.6024, -8.365) (-1.601, -8.3745) (-1.5996, -8.3841) (-1.5981, -8.3937) (-1.5966, -8.4035) (-1.5951, -8.4132) (-1.5935, -8.4231) (-1.5918, -8.433) (-1.5901, -8.443) (-1.5884, -8.453) (-1.5866, -8.4631) (-1.5848, -8.4733) (-1.5829, -8.4835) (-1.581, -8.4938) (-1.5791, -8.5041) (-1.577, -8.5145) (-1.575, -8.525) (-1.5729, -8.5355) (-1.5707, -8.546) (-1.5685, -8.5567) (-1.5663, -8.5673) (-1.564, -8.5781) (-1.5616, -8.5889) (-1.5592, -8.5997) (-1.5568, -8.6106) (-1.5543, -8.6215) (-1.5517, -8.6325) (-1.5492, -8.6436) (-1.5465, -8.6547) (-1.5438, -8.6659) (-1.5411, -8.6771) (-1.5383, -8.6883) (-1.5354, -8.6996) (-1.5325, -8.711) (-1.5296, -8.7224) (-1.5266, -8.7338) (-1.5235, -8.7453) (-1.5204, -8.7569) (-1.5173, -8.7684) (-1.514, -8.7801) (-1.5108, -8.7918) (-1.5075, -8.8035) (-1.5041, -8.8153) (-1.5007, -8.8271) (-1.4972, -8.8389) (-1.4937, -8.8508) (-1.4901, -8.8628) (-1.4865, -8.8747) (-1.4828, -8.8868) (-1.479, -8.8988) (-1.4752, -8.9109) (-1.4714, -8.9231) (-1.4675, -8.9353) (-1.4635, -8.9475) (-1.4595, -8.9598) (-1.4554, -8.9721) (-1.4513, -8.9844) (-1.4471, -8.9968) (-1.4429, -9.0092) (-1.4386, -9.0217) (-1.4343, -9.0342) (-1.4299, -9.0467) (-1.4254, -9.0593) (-1.4209, -9.0718) (-1.4163, -9.0845) (-1.4117, -9.0971) (-1.407, -9.1098) (-1.4023, -9.1226) (-1.3975, -9.1353) (-1.3927, -9.1481) (-1.3877, -9.161) (-1.3828, -9.1738) (-1.3778, -9.1867) (-1.3727, -9.1997) (-1.3676, -9.2126) (-1.3624, -9.2256) (-1.3571, -9.2386) (-1.3518, -9.2517) (-1.3465, -9.2647) (-1.3411, -9.2778) (-1.3356, -9.291) (-1.3301, -9.3041) (-1.3245, -9.3173) (-1.3188, -9.3305) (-1.3131, -9.3438) (-1.3074, -9.3571) (-1.3015, -9.3704) (-1.2957, -9.3837) (-1.2897, -9.397) (-1.2837, -9.4104) (-1.2777, -9.4238) (-1.2716, -9.4372) (-1.2654, -9.4507) (-1.2592, -9.4641) (-1.2529, -9.4776) (-1.2465, -9.4911) (-1.2401, -9.5047) (-1.2337, -9.5182) (-1.2272, -9.5318) (-1.2206, -9.5454) (-1.214, -9.559) (-1.2073, -9.5727) (-1.2005, -9.5863) (-1.1937, -9.6) (-1.1868, -9.6137) (-1.1799, -9.6275) (-1.1729, -9.6412) (-1.1659, -9.655) (-1.1588, -9.6687) (-1.1516, -9.6825) (-1.1444, -9.6964) (-1.1371, -9.7102) (-1.1298, -9.7241) (-1.1224, -9.7379) (-1.1149, -9.7518) (-1.1074, -9.7657) (-1.0998, -9.7796) (-1.0922, -9.7936) (-1.0845, -9.8075) (-1.0767, -9.8215) (-1.0689, -9.8355) (-1.061, -9.8494) (-1.0531, -9.8635) (-1.0451, -9.8775) (-1.037, -9.8915) (-1.0289, -9.9056) (-1.0207, -9.9196) (-1.0125, -9.9337) (-1.0042, -9.9478) (-0.9959, -9.9619) (-0.9875, -9.976) (-0.979, -9.9901) (-0.9705, -10.0042) (-0.9619, -10.0184) (-0.9532, -10.0325) (-0.9445, -10.0467) (-0.9357, -10.0608) (-0.9269, -10.075) (-0.918, -10.0892) (-0.9091, -10.1034) (-0.9001, -10.1176) (-0.891, -10.1318) (-0.8819, -10.1461) (-0.8727, -10.1603) (-0.8635, -10.1745) (-0.8542, -10.1888) (-0.8448, -10.203) (-0.8354, -10.2173) (-0.8259, -10.2316) (-0.8163, -10.2458) (-0.8067, -10.2601) (-0.7971, -10.2744) (-0.7874, -10.2887) (-0.7776, -10.303) (-0.7677, -10.3173) (-0.7578, -10.3316) (-0.7479, -10.3459) (-0.7399, -10.3573) (-0.7338, -10.3659) (-0.7298, -10.3716) (-0.7278, -10.3745) knots 0 0 0 0 0 0 0.00416667 0.00833333 0.0125 0.01666667 0.02083333 0.025 0.02916667 0.03333333 0.0375 0.04166667 0.04583333 0.05 0.05416667 0.05833333 0.0625 0.06666667 0.07083333 0.075 0.07916667 0.08333333 0.0875 0.09166667 0.09583333 0.1 0.10416667 0.10833333 0.1125 0.11666667 0.12083333 0.125 0.12916667 0.13333333 0.1375 0.14166667 0.14583333 0.15 0.15416667 0.15833333 0.1625 0.16666667 0.17083333 0.175 0.17916667 0.18333333 0.1875 0.19166667 0.19583333 0.2 0.20416667 0.20833333 0.2125 0.21666667 0.22083333 0.225 0.22916667 0.23333333 0.2375 0.24166667 0.24583333 0.25 0.25416667 0.25833333 0.2625 0.26666667 0.27083333 0.275 0.27916667 0.28333333 0.2875 0.29166667 0.29583333 0.3 0.30416667 0.30833333 0.3125 0.31666667 0.32083333 0.325 0.32916667 0.33333333 0.3375 0.34166667 0.34583333 0.35 0.35416667 0.35833333 0.3625 0.36666667 0.37083333 0.375 0.37916667 0.38333333 0.3875 0.39166667 0.39583333 0.4 0.40416667 0.40833333 0.4125 0.41666667 0.42083333 0.425 0.42916667 0.43333333 0.4375 0.44166667 0.44583333 0.45 0.45416667 0.45833333 0.4625 0.46666667 0.47083333 0.475 0.47916667 0.48333333 0.4875 0.49166667 0.49583333 0.5 0.50416667 0.50833333 0.5125 0.51666667 0.52083333 0.525 0.52916667 0.53333333 0.5375 0.54166667 0.54583333 0.55 0.55416667 0.55833333 0.5625 0.56666667 0.57083333 0.575 0.57916667 0.58333333 0.5875 0.59166667 0.59583333 0.6 0.60416667 0.60833333 0.6125 0.61666667 0.62083333 0.625 0.62916667 0.63333333 0.6375 0.64166667 0.64583333 0.65 0.65416667 0.65833333 0.6625 0.66666667 0.67083333 0.675 0.67916667 0.68333333 0.6875 0.69166667 0.69583333 0.7 0.70416667 0.70833333 0.7125 0.71666667 0.72083333 0.725 0.72916667 0.73333333 0.7375 0.74166667 0.74583333 0.75 0.75416667 0.75833333 0.7625 0.76666667 0.77083333 0.775 0.77916667 0.78333333 0.7875 0.79166667 0.79583333 0.8 0.80416667 0.80833333 0.8125 0.81666667 0.82083333 0.825 0.82916667 0.83333333 0.8375 0.84166667 0.84583333 0.85 0.85416667 0.85833333 0.8625 0.86666667 0.87083333 0.875 0.87916667 0.88333333 0.8875 0.89166667 0.89583333 0.9 0.90416667 0.90833333 0.9125 0.91666667 0.92083333 0.925 0.92916667 0.93333333 0.9375 0.94166667 0.94583333 0.95 0.95416667 0.95833333 0.9625 0.96666667 0.97083333 0.975 0.97916667 0.98333333 0.9875 0.99166667 0.99583333 1 1 1 1 1 1
  arc A5 (-0.7278, -10.3745) -> (0.7278, -10.3745) centre (0, 0) ccw
  spline S5 degree 5 poles (0.7278, -10.3745) (0.7298, -10.3716) (0.7338, -10.3659) (0.7399, -10.3573) (0.7479, -10.3459) (0.7578, -10.3316) (0.7677, -10.3173) (0.7776, -10.303) (0.7874, -10.2887) (0.7971, -10.2744) (0.8067, -10.2601) (0.8163, -10.2458) (0.8259, -10.2316) (0.8354, -10.2173) (0.8448, -10.203) (0.8542, -10.1888) (0.8635, -10.1745) (0.8727, -10.1603) (0.8819, -10.1461) (0.891, -10.1318) (0.9001, -10.1176) (0.9091, -10.1034) (0.918, -10.0892) (0.9269, -10.075) (0.9357, -10.0608) (0.9445, -10.0467) (0.9532, -10.0325) (0.9619, -10.0184) (0.9705, -10.0042) (0.979, -9.9901) (0.9875, -9.976) (0.9959, -9.9619) (1.0042, -9.9478) (1.0125, -9.9337) (1.0207, -9.9196) (1.0289, -9.9056) (1.037, -9.8915) (1.0451, -9.8775) (1.0531, -9.8635) (1.061, -9.8494) (1.0689, -9.8355) (1.0767, -9.8215) (1.0845, -9.8075) (1.0922, -9.7936) (1.0998, -9.7796) (1.1074, -9.7657) (1.1149, -9.7518) (1.1224, -9.7379) (1.1298, -9.7241) (1.1371, -9.7102) (1.1444, -9.6964) (1.1516, -9.6825) (1.1588, -9.6687) (1.1659, -9.655) (1.1729, -9.6412) (1.1799, -9.6275) (1.1868, -9.6137) (1.1937, -9.6) (1.2005, -9.5863) (1.2073, -9.5727) (1.214, -9.559) (1.2206, -9.5454) (1.2272, -9.5318) (1.2337, -9.5182) (1.2401, -9.5047) (1.2465, -9.4911) (1.2529, -9.4776) (1.2592, -9.4641) (1.2654, -9.4507) (1.2716, -9.4372) (1.2777, -9.4238) (1.2837, -9.4104) (1.2897, -9.397) (1.2957, -9.3837) (1.3015, -9.3704) (1.3074, -9.3571) (1.3131, -9.3438) (1.3188, -9.3305) (1.3245, -9.3173) (1.3301, -9.3041) (1.3356, -9.291) (1.3411, -9.2778) (1.3465, -9.2647) (1.3518, -9.2517) (1.3571, -9.2386) (1.3624, -9.2256) (1.3676, -9.2126) (1.3727, -9.1997) (1.3778, -9.1867) (1.3828, -9.1738) (1.3877, -9.161) (1.3927, -9.1481) (1.3975, -9.1353) (1.4023, -9.1226) (1.407, -9.1098) (1.4117, -9.0971) (1.4163, -9.0845) (1.4209, -9.0718) (1.4254, -9.0593) (1.4299, -9.0467) (1.4343, -9.0342) (1.4386, -9.0217) (1.4429, -9.0092) (1.4471, -8.9968) (1.4513, -8.9844) (1.4554, -8.9721) (1.4595, -8.9598) (1.4635, -8.9475) (1.4675, -8.9353) (1.4714, -8.9231) (1.4752, -8.9109) (1.479, -8.8988) (1.4828, -8.8868) (1.4865, -8.8747) (1.4901, -8.8628) (1.4937, -8.8508) (1.4972, -8.8389) (1.5007, -8.8271) (1.5041, -8.8153) (1.5075, -8.8035) (1.5108, -8.7918) (1.514, -8.7801) (1.5173, -8.7684) (1.5204, -8.7569) (1.5235, -8.7453) (1.5266, -8.7338) (1.5296, -8.7224) (1.5325, -8.711) (1.5354, -8.6996) (1.5383, -8.6883) (1.5411, -8.6771) (1.5438, -8.6659) (1.5465, -8.6547) (1.5492, -8.6436) (1.5517, -8.6325) (1.5543, -8.6215) (1.5568, -8.6106) (1.5592, -8.5997) (1.5616, -8.5889) (1.564, -8.5781) (1.5663, -8.5673) (1.5685, -8.5567) (1.5707, -8.546) (1.5729, -8.5355) (1.575, -8.525) (1.577, -8.5145) (1.5791, -8.5041) (1.581, -8.4938) (1.5829, -8.4835) (1.5848, -8.4733) (1.5866, -8.4631) (1.5884, -8.453) (1.5901, -8.443) (1.5918, -8.433) (1.5935, -8.4231) (1.5951, -8.4132) (1.5966, -8.4035) (1.5981, -8.3937) (1.5996, -8.3841) (1.601, -8.3745) (1.6024, -8.365) (1.6037, -8.3555) (1.605, -8.3461) (1.6062, -8.3368) (1.6074, -8.3276) (1.6086, -8.3184) (1.6097, -8.3093) (1.6108, -8.3002) (1.6118, -8.2913) (1.6128, -8.2824) (1.6138, -8.2735) (1.6147, -8.2648) (1.6156, -8.2561) (1.6164, -8.2475) (1.6172, -8.239) (1.618, -8.2306) (1.6187, -8.2222) (1.6194, -8.2139) (1.6201, -8.2057) (1.6207, -8.1976) (1.6213, -8.1895) (1.6218, -8.1815) (1.6223, -8.1737) (1.6228, -8.1658) (1.6233, -8.1581) (1.6237, -8.1505) (1.6241, -8.143) (1.6244, -8.1355) (1.6247, -8.1281) (1.625, -8.1208) (1.6253, -8.1136) (1.6255, -8.1065) (1.6257, -8.0995) (1.6258, -8.0926) (1.626, -8.0858) (1.6261, -8.079) (1.6262, -8.0724) (1.6262, -8.0659) (1.6263, -8.0594) (1.6263, -8.0531) (1.6262, -8.0468) (1.6262, -8.0407) (1.6261, -8.0346) (1.626, -8.0287) (1.6259, -8.0229) (1.6258, -8.0171) (1.6257, -8.0115) (1.6255, -8.006) (1.6253, -8.0006) (1.6251, -7.9953) (1.6249, -7.9901) (1.6246, -7.985) (1.6244, -7.9801) (1.6241, -7.9752) (1.6238, -7.9705) (1.6235, -7.9659) (1.6232, -7.9614) (1.6229, -7.957) (1.6226, -7.9528) (1.6223, -7.9487) (1.6219, -7.9447) (1.6216, -7.9408) (1.6212, -7.9371) (1.6209, -7.9334) (1.6205, -7.93) (1.6202, -7.9266) (1.6198, -7.9234) (1.6195, -7.9204) (1.6191, -7.9174) (1.6188, -7.9146) (1.6184, -7.912) (1.6181, -7.9095) (1.6178, -7.9072) (1.6175, -7.905) (1.6172, -7.9029) (1.6169, -7.9011) (1.6166, -7.8993) (1.6164, -7.8978) (1.6161, -7.8964) (1.6159, -7.8951) (1.6157, -7.8941) (1.6156, -7.8933) (1.6155, -7.8929) (1.6155, -7.8926) (1.6154, -7.8925) knots -1 -1 -1 -1 -1 -1 -0.99583333 -0.99166667 -0.9875 -0.98333333 -0.97916667 -0.975 -0.97083333 -0.96666667 -0.9625 -0.95833333 -0.95416667 -0.95 -0.94583333 -0.94166667 -0.9375 -0.93333333 -0.92916667 -0.925 -0.92083333 -0.91666667 -0.9125 -0.90833333 -0.90416667 -0.9 -0.89583333 -0.89166667 -0.8875 -0.88333333 -0.87916667 -0.875 -0.87083333 -0.86666667 -0.8625 -0.85833333 -0.85416667 -0.85 -0.84583333 -0.84166667 -0.8375 -0.83333333 -0.82916667 -0.825 -0.82083333 -0.81666667 -0.8125 -0.80833333 -0.80416667 -0.8 -0.79583333 -0.79166667 -0.7875 -0.78333333 -0.77916667 -0.775 -0.77083333 -0.76666667 -0.7625 -0.75833333 -0.75416667 -0.75 -0.74583333 -0.74166667 -0.7375 -0.73333333 -0.72916667 -0.725 -0.72083333 -0.71666667 -0.7125 -0.70833333 -0.70416667 -0.7 -0.69583333 -0.69166667 -0.6875 -0.68333333 -0.67916667 -0.675 -0.67083333 -0.66666667 -0.6625 -0.65833333 -0.65416667 -0.65 -0.64583333 -0.64166667 -0.6375 -0.63333333 -0.62916667 -0.625 -0.62083333 -0.61666667 -0.6125 -0.60833333 -0.60416667 -0.6 -0.59583333 -0.59166667 -0.5875 -0.58333333 -0.57916667 -0.575 -0.57083333 -0.56666667 -0.5625 -0.55833333 -0.55416667 -0.55 -0.54583333 -0.54166667 -0.5375 -0.53333333 -0.52916667 -0.525 -0.52083333 -0.51666667 -0.5125 -0.50833333 -0.50416667 -0.5 -0.49583333 -0.49166667 -0.4875 -0.48333333 -0.47916667 -0.475 -0.47083333 -0.46666667 -0.4625 -0.45833333 -0.45416667 -0.45 -0.44583333 -0.44166667 -0.4375 -0.43333333 -0.42916667 -0.425 -0.42083333 -0.41666667 -0.4125 -0.40833333 -0.40416667 -0.4 -0.39583333 -0.39166667 -0.3875 -0.38333333 -0.37916667 -0.375 -0.37083333 -0.36666667 -0.3625 -0.35833333 -0.35416667 -0.35 -0.34583333 -0.34166667 -0.3375 -0.33333333 -0.32916667 -0.325 -0.32083333 -0.31666667 -0.3125 -0.30833333 -0.30416667 -0.3 -0.29583333 -0.29166667 -0.2875 -0.28333333 -0.27916667 -0.275 -0.27083333 -0.26666667 -0.2625 -0.25833333 -0.25416667 -0.25 -0.24583333 -0.24166667 -0.2375 -0.23333333 -0.22916667 -0.225 -0.22083333 -0.21666667 -0.2125 -0.20833333 -0.20416667 -0.2 -0.19583333 -0.19166667 -0.1875 -0.18333333 -0.17916667 -0.175 -0.17083333 -0.16666667 -0.1625 -0.15833333 -0.15416667 -0.15 -0.14583333 -0.14166667 -0.1375 -0.13333333 -0.12916667 -0.125 -0.12083333 -0.11666667 -0.1125 -0.10833333 -0.10416667 -0.1 -0.09583333 -0.09166667 -0.0875 -0.08333333 -0.07916667 -0.075 -0.07083333 -0.06666667 -0.0625 -0.05833333 -0.05416667 -0.05 -0.04583333 -0.04166667 -0.0375 -0.03333333 -0.02916667 -0.025 -0.02083333 -0.01666667 -0.0125 -0.00833333 -0.00416667 0 0 0 0 0 0
  line L10 (1.6154, -7.8925) -> (1.6152, -7.8914)
  line L11 (1.6152, -7.8914) -> (1.147, -5.6038)
  arc A6 (1.147, -5.6038) -> (3.1514, -4.7736) centre (0, 0) ccw
  line L12 (3.1514, -4.7736) -> (4.4379, -6.7222)
  line L13 (4.4379, -6.7222) -> (4.4385, -6.7231)